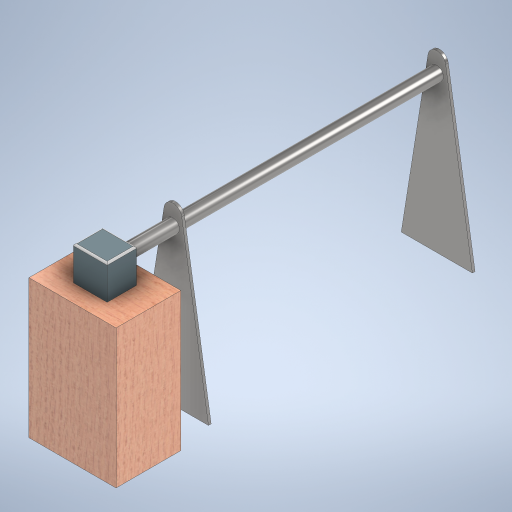
# Autodesk Inventor part: stand
Saved by Autodesk Inventor 2024 (Build 280153000, 153)
## iProperties
Created: 2024-01-19
Part Number: stand
Material: Generic
Document SubType Name: Modeling
Designer: HP
Density: 1 g/cm^3
Appearance: Default
Author: HP
Autodesk Inventor part; units mm, degrees
ref_plane "YZ Plane" through (0, 0, 0) normal (1, 0, 0) x (0, 1, 0)
ref_plane "XZ Plane" through (0, 0, 0) normal (0, 1, 0) x (-1, 0, 0)
ref_plane "XY Plane" through (0, 0, 0) normal (0, 0, 1) x (1, 0, 0)
sketch "Sketch1" plane through (0, 0, 0) normal (0, 0, 1) x (1, 0, 0)
  point P0 (0, 0)
sketch "Sketch2" plane through (0, 0, 0) normal (0, 0, 1) x (1, 0, 0)
  line L0 (0, 0) -> (80, 0)
  line L1 (80, 0) -> (40, 250)
  line L2 (40, 250) -> (0, 0)
  dimension "d0" = 80
  dimension "d1" = 250
  dimension "d2" = 40
  constraints: 6 end point, 1 horizontal
  measures "d0" distance of L0.start L0.end
  measures "d1" distance from line of L0 L1.end
  measures "d2" horizontal distance of L0.start L1.end
extrude "Extrusion1" add sketch "Sketch2" against normal blind 3
sketch "Sketch3" plane through (0, 0, -3) normal (0, 0, -1) x (-1, 0, 0)
  circle A0 centre (-40, 175) radius 7.5
  line L0 (-80, 0) -> (0, 0) projected
  point P0 (-40, 250)
  point P1 (-40, 0)
  dimension "d5" = 15
  dimension "d6" = 0
  dimension "d7" = 175
  constraints: 1 centre point, 1 midpoint
  measures "d5" diameter of A0
  measures "d6" horizontal distance of point (-40, 250) A0.centre
  measures "d7" distance of point (-40, 0) A0.centre
fillet "Fillet1" radius 10 1 edges at (40, 250, -1.5)
extrude "Extrusion2" add sketch "Sketch3" along normal blind 147
mirror "Mirror1" about plane through (40, 175, -150) normal (0, 0, -1) of "Extrusion2", "Extrusion1"
fillet "Fillet2" radius 10 1 edges at (40, 250, -298.5)
sketch "Sketch4" plane through (0, 0, 0) normal (0, 0, 1) x (1, 0, 0)
  circle A0 centre (40, 175) radius 7.5 projected
  circle A1 centre (40, 175) radius 7.5
  point P0 (0, 0)
  constraints: 1 centre point, 1 coincident
extrude "Extrusion3" add sketch "Sketch4" along normal blind 50
sketch "Sketch5" plane through (40, 175, 50) normal (0, 0, 1) x (1, 0, 0)
  circle A0 centre (0, 0) radius 2.5
  point P0 (-40, -175)
  dimension "d14" = 5
  constraints: 1 centre point
  measures "d14" diameter of A0
extrude "Extrusion4" add sketch "Sketch5" along normal blind 10
sketch "Sketch6" plane through (40, 175, 60) normal (0, 0, 1) x (1, 0, 0)
  line L0 (-19, 19) -> (19, 19)
  line L1 (19, 19) -> (19, -19)
  line L2 (19, -19) -> (-19, -19)
  line L3 (-19, -19) -> (-19, 19)
  circle A0 centre (0, 0) radius 2.5 projected
  point P0 (-40, -175)
  dimension "d17" = 38
  dimension "d18" = 38
  dimension "d19" = 19
  dimension "d20" = 19
  constraints: 8 end point, 2 parallel, 1 horizontal, 1 perpendicular
  measures "d17" distance of L0.end L1.end
  measures "d18" distance of L0.start L0.end
  measures "d19" distance from line of A0.centre L1
  measures "d20" distance from line of A0.centre L0
extrude "Extrusion5" add sketch "Sketch6" along normal blind 33 contours L0 L1 L2 L3 | A0
sketch "Sketch7" plane through (21, 156, 60) normal (0, -1, 0) x (1, 0, 0)
  line L0 (-30, 53) -> (68, 53)
  line L1 (68, 53) -> (68, -20)
  line L2 (68, -20) -> (-30, -20)
  line L3 (-30, -20) -> (-30, 53)
  line L4 (38, 0) -> (38, 33) projected
  line L5 (0, 0) -> (0, 33) projected
  line L6 (0, 33) -> (38, 33) projected
  point P0 (-21, -60)
  point P1 (38, 16.5)
  point P2 (68, 16.5)
  point P3 (-30, 16.5)
  point P4 (0, 16.5)
  dimension "d23" = 30
  dimension "d24" = 30
  dimension "d25" = 20
  dimension "d26" = 20
  constraints: 8 end point, 4 midpoint, 2 parallel, 1 horizontal, 1 perpendicular
  measures "d23" distance of point (38, 16.5) point (68, 16.5)
  measures "d24" distance of point (-30, 16.5) point (0, 16.5)
  measures "d25" distance from line of L4.start L2
  measures "d26" distance between parallel lines of L0 L6
extrude "Extrusion6" add sketch "Sketch7" along normal blind 156
fillet "Fillet3" radius 2 4 edges at (21, 194, 76.5) (59, 194, 76.5) (40, 194, 60) (40, 194, 93)
body "Solid1"
